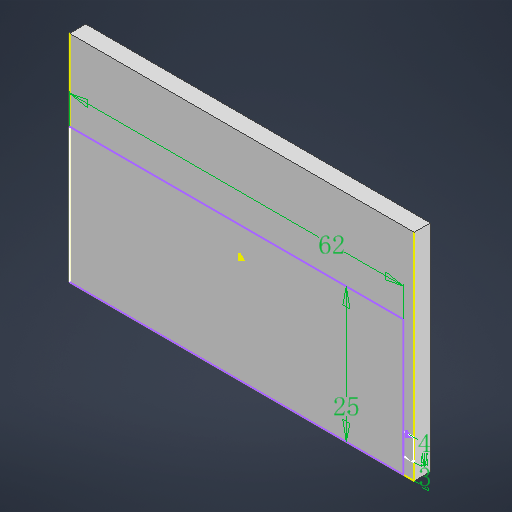
# Autodesk Inventor part: 摄像头电路部分
Saved by Autodesk Inventor 2025 (Build 290162000, 162)
## iProperties
Created: 2025-10-27
Part Number: 摄像头电路部分
Material: 常规
Document SubType Name: Modeling
Designer: XH
Density: 1 g/cm^3
Appearance: 默认
Author: XH
Autodesk Inventor part; units mm, degrees
ref_plane "YZ Plane" through (0, 0, 0) normal (1, 0, 0) x (0, 1, 0)
ref_plane "XZ Plane" through (0, 0, 0) normal (0, 1, 0) x (-1, 0, 0)
ref_plane "XY Plane" through (0, 0, 0) normal (0, 0, 1) x (1, 0, 0)
sketch "草图1" plane through (0, 0, 0) normal (0, 0, 1) x (1, 0, 0)
  line L0 (32, -20) -> (-32, -20)
  line L1 (-32, -20) -> (-32, 20)
  line L2 (-32, 20) -> (32, 20)
  line L3 (32, 20) -> (32, -20)
  line L4 (32, -20) -> (-32, 20) construction
  line L5 (-32, -20) -> (32, 20) construction
  line L6 (-32, 10) -> (-30, 10)
  line L7 (-30, 10) -> (-30, -20)
  line L8 (-30, -20) -> (-32, -20)
  line L9 (-32, -20) -> (-32, 10)
  point P0 (0, 0)
  dimension "d0" = 64
  dimension "d1" = 40
  dimension "d2" = 2
  dimension "d3" = 30
  constraints: 20 end point, 4 parallel, 2 horizontal, 2 midpoint, 2 perpendicular, 2 point on line
  measures "d0" distance of L1.end L2.end
  measures "d1" distance of L0.end L1.end
  measures "d2" distance between parallel lines of L1 L7
  measures "d3" distance between parallel lines of L0 L6
extrude "拉伸1" add sketch "草图1" along normal blind 3
sketch "草图2" plane through (0, 0, 3) normal (0, 0, 1) x (1, 0, 0)
  line L0 (-32, -20) -> (30, -20)
  line L1 (30, 5) -> (-32, 5)
  line L2 (-32, 5) -> (-32, -20)
  line L3 (-32, 20) -> (-32, -20) projected
  line L4 (32, -20) -> (32, 20) projected
  line L5 (30, -13) -> (32, -13)
  line L6 (32, -13) -> (32, -17)
  line L7 (32, -17) -> (30, -17)
  line L8 (30, -17) -> (30, -13)
  line L9 (-32, -20) -> (32, -20) projected
  line L10 (30, 5) -> (30, -20)
  point P0 (0, 0)
  point P1 (31, -13)
  dimension "d6" = 62
  dimension "d7" = 4
  dimension "d8" = 3
  dimension "d9" = 25
  constraints: 16 end point, 2 parallel, 1 collinear, 1 horizontal, 1 midpoint, 1 perpendicular, 1 point on line, 1 vertical
  measures "d6" distance of L1.start L1.end
  measures "d7" distance from line of point (31, -13) L7
  measures "d8" distance between parallel lines of L7 L9
  measures "d9" distance between parallel lines of L0 L1
